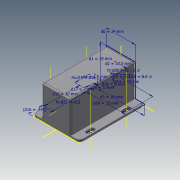
# Autodesk Inventor part: ADAFRUIT 1512 LOCK SOLENOID
Saved by Autodesk Inventor 2020.3 (Build 243373000, 373)
## iProperties
RuleStatus: InUse
AfterDocSave0: file://Part Number Cleaner
Created: 2020-01-27
Material: Generic
Vendor: HHMI: JRC - ID&F
Document SubType Name: Modeling
Designer: arnoldj
Density: 1 g/cm^3
Appearance: Default
DESIGN DEPARTMENT: HHMI: JRC - ID&F
ALTERED ITEM PART NUMBER: N/A
ALTERED ITEM VENDOR: N/A
ALTERED ITEM DESCRIPTION: N/A
Author: arnoldj
Revision Number: 0
Autodesk Inventor part; units mm, degrees
ref_plane "YZ Plane" through (0, 0, 0) normal (1, 0, 0) x (0, 1, 0)
ref_plane "XZ Plane" through (0, 0, 0) normal (0, 1, 0) x (-1, 0, 0)
ref_plane "XY Plane" through (0, 0, 0) normal (0, 0, 1) x (1, 0, 0)
sketch "Sketch1" plane through (0, 0, 0) normal (0, 0, 1) x (1, 0, 0)
  line L0 (0, 33.6) -> (0, -5.6) projected
  line L1 (-27.3, 0) -> (27.3, 0) projected
  line L2 (12, 28) -> (-12, 28)
  line L3 (-12, 28) -> (-12, 0)
  line L4 (-12, 0) -> (12, 0)
  line L5 (12, 0) -> (12, 28)
  line L6 (12, 28) -> (-12, 0) construction
  line L7 (-12, 28) -> (12, 0) construction
  line L8 (5.25, 8) -> (-5.25, 8)
  line L9 (-5.25, 8) -> (-5.25, 18.5)
  line L10 (-5.25, 18.5) -> (5.25, 18.5)
  line L11 (5.25, 18.5) -> (5.25, 8)
  line L12 (-12, 0) -> (-19.5, 0)
  line L13 (-19.5, 0) -> (-19.5, 1.5)
  line L14 (-19.5, 1.5) -> (-12, 1.5)
  line L15 (-12, 1.5) -> (-12, 0)
  line L16 (12, 0) -> (19.5, 0)
  line L17 (19.5, 0) -> (19.5, 1.5)
  line L18 (19.5, 1.5) -> (12, 1.5)
  line L19 (12, 1.5) -> (12, 0)
  circle A0 centre (0, 13.25) radius 10.16
  line L20 (-5.25, 18.5) -> (5.25, 8) construction
  line L21 (5.25, 18.5) -> (-5.25, 8) construction
  point P0 (0, 0)
  point P1 (0, 13.25)
  point P2 (0, 13.25)
  dimension "d0" = 24
  dimension "d1" = 28
  dimension "d2" = 10.5
  dimension "d3" = 39
  dimension "d4" = 1.5
  dimension "d10" = 20.32
  dimension "d30" = 5.25
  dimension "d32" = 0
  dimension "d35" = 8
  constraints: 40 end point, 8 parallel, 4 horizontal, 4 perpendicular, 2 coincident, 2 equal length, 2 midpoint, 2 point on line, 1 centre point
  measures "d0" distance of L2.start L2.end
  measures "d1" distance of L2.end L3.end
  measures "d2" distance of L9.end L10.end
  measures "d3" distance of L17.end L13.end
  measures "d4" distance of L12.end L13.end
  measures "d10" diameter of A0
  measures "d30" distance between parallel lines of L0 L11
  measures "d32" distance of point (0, 13.25) point (0, 13.25)
  measures "d35" distance between parallel lines of L4 L8
extrude "Extrusion1" add sketch "Sketch1" along normal blind 54
extrude "Extrusion3" add sketch "Sketch1" against normal blind 1 contours A0 L0 L8 L11 L10 | L0 L10 L9 L8 A0
sketch "Sketch3" plane through (-19.5, 0, 0) normal (0, -1, 0) x (1, 0, 0)
  line L0 (19.5, 64.8) -> (19.5, -10.8) projected
  line L1 (-7.8, 0) -> (46.8, 0) projected
  line L2 (0, 54) -> (39, 54) projected
  line L3 (36, 42) -> (3, 42) construction
  line L4 (3, 42) -> (3, 12) construction
  line L5 (3, 12) -> (36, 12) construction
  line L6 (36, 12) -> (36, 42) construction
  line L7 (36, 42) -> (3, 12) construction
  line L8 (3, 42) -> (36, 12) construction
  line L9 (3, 14) -> (3, 10) construction
  line L10 (4.5, 14) -> (4.5, 10)
  line L11 (1.5, 10) -> (1.5, 14)
  arc A0 (4.5, 14) -> (1.5, 14) centre (3, 14) ccw
  arc A1 (1.5, 10) -> (4.5, 10) centre (3, 10) ccw
  arc A2 (4.5, 44) -> (1.5, 44) centre (3, 44) ccw
  line L12 (4.5, 44) -> (4.5, 40)
  line L13 (3, 44) -> (3, 40) construction
  line L14 (1.5, 40) -> (1.5, 44)
  arc A3 (1.5, 40) -> (4.5, 40) centre (3, 40) ccw
  arc A4 (37.5, 14) -> (34.5, 14) centre (36, 14) ccw
  line L15 (37.5, 14) -> (37.5, 10)
  line L16 (36, 14) -> (36, 10) construction
  line L17 (34.5, 10) -> (34.5, 14)
  arc A5 (34.5, 10) -> (37.5, 10) centre (36, 10) ccw
  arc A6 (37.5, 44) -> (34.5, 44) centre (36, 44) ccw
  line L18 (37.5, 44) -> (37.5, 40)
  line L19 (36, 44) -> (36, 40) construction
  line L20 (34.5, 40) -> (34.5, 44)
  arc A7 (34.5, 40) -> (37.5, 40) centre (36, 40) ccw
  point P0 (19.5, 0)
  point P1 (19.5, 27)
  dimension "d13" = 30
  dimension "d14" = 33
  dimension "d15" = 12
  dimension "d16" = 12
  dimension "d17" = 7
  dimension "d18" = 3
  dimension "d21" = 30
  dimension "d24" = 33
  constraints: 44 end point, 16 point on circle, 8 centre point, 7 coincident, 4 midpoint, 4 tangent, 3 parallel, 2 horizontal, 2 vertical, 1 perpendicular, 39 other
  measures "d13" distance of L3.end L4.end
  measures "d14" distance of L4.end L5.end
  measures "d15" distance between parallel lines of L5 L1
  measures "d16" distance between parallel lines of L2 L3
  measures "d18" distance between parallel lines of L10 L11
  measures "d21" distance of L10.start L12.start
  measures "d24" distance of L10.start L15.start
extrude "Extrusion4" cut sketch "Sketch3" against normal up to next
fillet "Fillet1" radius 3.175 4 edges at (-19.5, 0.75, 0) (-19.5, 0.75, 54) (19.5, 0.75, 0) (19.5, 0.75, 54)
fillet "Fillet2" radius 1.27 4 edges at (-12, 14.75, 0) (12, 14.75, 0) (-12, 14.75, 54) (12, 14.75, 54)
fillet "Fillet3" radius 1.27 11 edges at (-12, 28, 27) (-12, 1.5, 27) (-11.628, 28, 53.628) (0, 28, 54) (11.628, 28, 53.628) (12, 28, 27) (11.628, 28, 0.372) (0, 28, 0) (-11.628, 28, 0.372) (-11.628, 1.5, 53.628) (-11.628, 1.5, 0.372)
equation "\"d30\" = 0.5 * d2"
equation "\"d15\" = d16"
equation "\"d21\" = d13"
body "Solid1"
